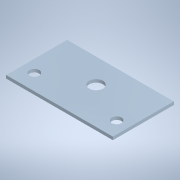
# Autodesk Inventor part: CLS_typeC_31.4N_plate
Saved by Autodesk Inventor 2021.3 (Build 253353010, 353A)
## iProperties
Created: 2021-01-11
Part Number: CLS_typeC_31.4N_plate
Material: 一般
Document SubType Name: Modeling
Designer: YusukeKunita
Density: 1 g/cm^3
Appearance: 鋼色
Author: YusukeKunita
Autodesk Inventor part; units mm, degrees
ref_plane "YZ Plane" through (0, 0, 0) normal (1, 0, 0) x (0, 1, 0)
ref_plane "XZ Plane" through (0, 0, 0) normal (0, 1, 0) x (-1, 0, 0)
ref_plane "XY Plane" through (0, 0, 0) normal (0, 0, 1) x (1, 0, 0)
sketch "スケッチ1" plane through (0, 0, 0) normal (0, 0, 1) x (1, 0, 0)
  line L0 (0, 0) -> (35, 0)
  line L1 (35, 0) -> (35, 20)
  line L2 (35, 20) -> (0, 20)
  line L3 (0, 20) -> (0, 0)
  dimension "d0" = 20
  dimension "d1" = 35
  constraints: 8 end point, 2 parallel, 1 horizontal, 1 perpendicular
  measures "d0" distance of L0.end L1.end
  measures "d1" distance of L1.end L2.end
extrude "押し出し1" add sketch "スケッチ1" along normal blind 1
sketch "スケッチ2" plane through (0, 0, 1) normal (0, 0, 1) x (1, 0, 0)
  line L0 (35, 20) -> (0, 20) projected
  point P0 (0, 0)
  point P1 (17.5, 12)
  point P2 (17.5, 20)
  dimension "d4" = 8
  constraints: 1 midpoint, 1 vertical alignment
  measures "d4" distance from line of L0 point (17.5, 12)
hole "穴1" at (17.5, 12, 1) direction (0, 0, -1) diameter 4.5 end through all
sketch "スケッチ3" plane through (0, 0, 1) normal (0, 0, 1) x (1, 0, 0)
  line L0 (0, 20) -> (0, 0) projected
  line L1 (0, 0) -> (35, 0) projected
  line L2 (35, 20) -> (0, 20) projected
  point P0 (4, 5.25)
  point P1 (31, 5.25)
  dimension "d12" = 27
  dimension "d13" = 4
  dimension "d22" = 14.75
  constraints: 1 horizontal alignment
  measures "d12" distance of point (31, 5.25) point (4, 5.25)
  measures "d13" distance from line of L0 point (4, 5.25)
  measures "d22" distance from line of L2 point (31, 5.25)
hole "穴2" at (4, 5.25, 1) at (31, 5.25, 1) direction (0, 0, -1) diameter 3.2 end through all
